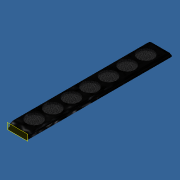
# Autodesk Inventor part: base
Saved by Autodesk Inventor 2015 (Build 190159000, 159)
## iProperties
Created: 2019-01-05
Part Number: base
Material: Generic
Document SubType Name: Modeling
Designer: gabriel
Density: 1 g/cm^3
Appearance: Default
Author: gabriel
Autodesk Inventor part; units mm, degrees
ref_plane "YZ Plane" through (0, 0, 0) normal (1, 0, 0) x (0, 1, 0)
ref_plane "XZ Plane" through (0, 0, 0) normal (0, 1, 0) x (-1, 0, 0)
ref_plane "XY Plane" through (0, 0, 0) normal (0, 0, 1) x (1, 0, 0)
sketch "Sketch16" plane through (0, 0, 0) normal (0, 0, 1) x (1, 0, 0)
  line L0 (0, 0) -> (-15.875, 0)
  line L1 (-15.875, -4.7625) -> (0, -4.7625)
  line L2 (0, 0) -> (0, -4.7625)
  line L3 (-15.875, -4.7625) -> (-15.875, 0)
  dimension "d96" = 15.875
  dimension "d184" = 4.7625
  constraints: 8 end point, 2 horizontal, 2 vertical
  measures "d96" distance of L0.start L0.end
  measures "d184" distance between parallel lines of L0 L1
extrude "Extrusion17" add sketch "Sketch16" along normal blind 114.3
sketch "Sketch17" plane through (-15.875, 0, 0) normal (0, 1, 0) x (1, 0, 0)
  circle A0 centre (7.9375, -104.775) radius 6.5768
  line L0 (0, 0) -> (0, -114.3) projected
  line L1 (15.875, -114.3) -> (0, -114.3) projected
  circle A1 centre (7.9375, -88.9) radius 6.5768
  circle A2 centre (7.9375, -73.025) radius 6.5768
  circle A3 centre (7.9375, -57.15) radius 6.5768
  circle A4 centre (7.9375, -41.275) radius 6.5768
  circle A5 centre (7.9375, -25.4) radius 6.5768
  circle A6 centre (7.9375, -9.525) radius 6.5768
  point P0 (15.875, 0)
  dimension "d102" = 13.1536
  dimension "d103" = 7.9375
  dimension "d104" = 9.525
  dimension "d107" = 15.875
  constraints: 7 centre point, 1 vertical, 12 other
  measures "d102" diameter of A0
  measures "d103" distance from line of L0 A0.centre
  measures "d104" distance from line of L1 A0.centre
  measures "d107" distance of A0.centre A1.centre
sketch "Sketch44" plane through (0, -4.7625, 0) normal (1, 0, 0) x (0, 0, -1)
  arc A0 (4.7625, 0) -> (0, 4.7625) centre (0, 0) ccw
  line L0 (0, 0) -> (4.7625, 0)
  line L1 (0, 4.7625) -> (0, 0)
  arc A1 (-114.3, 4.7625) -> (-119.0625, 0) centre (-114.3, 0) ccw
  line L2 (-114.3, 4.7625) -> (-114.3, 0)
  line L3 (-114.3, 0) -> (-119.0625, 0)
  constraints: 8 end point, 4 point on circle, 2 centre point, 2 perpendicular, 1 horizontal, 1 vertical
extrude "Extrusion40" add sketch "Sketch44" against normal up to surface (15.875 mm away)
ref_plane "Work Plane1" through (0, -4.7625, 119.0625) normal (0, 0, 1) x (1, 0, 0)
sketch "Sketch45" plane through (0, -4.7625, 119.0625) normal (0, 0, 1) x (1, 0, 0)
  line L0 (-15.875, 0) -> (-15.875, 4.7625) projected
  arc A0 (-15.875, 1.5875) -> (-15.875, 3.175) centre (-15.875, 2.3812) ccw
  line L1 (0, 4.7625) -> (0, 0) projected
  arc A1 (0, 3.175) -> (0, 1.5875) centre (0, 2.3813) ccw
  line L2 (-15.875, 3.175) -> (-15.875, 1.5875)
  line L3 (0, 3.175) -> (0, 1.5875)
  line L4 (0, 4.7625) -> (-15.875, 4.7625) projected
  dimension "d240" = 0.7937
  dimension "d241" = 0.7937
  dimension "d242" = 2.3813
  dimension "d243" = 2.3813
  constraints: 4 end point, 4 point on circle, 3 point on line, 2 centre point, 2 collinear, 2 midpoint
  measures "d240" radius of A0
  measures "d241" radius of A1
  measures "d242" distance from line of L4 A0.centre
  measures "d243" distance from line of L4 A1.centre
extrude "Extrusion41" cut sketch "Sketch45" against normal through all
extrude "Extrusion42" cut sketch "Sketch17" against normal blind 1.7859
body "Solid7"
